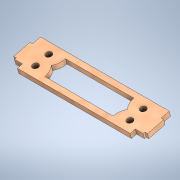
# Autodesk Inventor part: motor_holder
Saved by Autodesk Inventor 2022 (Build 260153070, 153G)
## iProperties
Created: 2021-05-28
Part Number: motor_holder
Material: Plywood, Sheathing, Glazed
Document SubType Name: Modeling
Designer: kardo
Density: 0.75 g/cm^3
Appearance: Plywood - New(2)
Author: kardo
Autodesk Inventor part; units mm, degrees
ref_plane "YZ Plane" through (0, 0, 0) normal (1, 0, 0) x (0, 1, 0)
ref_plane "XZ Plane" through (0, 0, 0) normal (0, 1, 0) x (-1, 0, 0)
ref_plane "XY Plane" through (0, 0, 0) normal (0, 0, 1) x (1, 0, 0)
derived "frame_outline.ipt"
sketch "motor_holder" plane through (6.24, -155.2, 37.8624) normal (0, 0.9709921, 0.2391117) x (-1, 0, 0)
  line L0 (-48.76, 5.318) -> (-48.76, -7.3978)
  line L1 (6.24, -320.5362) -> (6.24, 745.7309) construction
  line L2 (-48.76, 11.6759) -> (0.24, 11.6759)
  line L3 (-48.76, -13.7557) -> (0.24, -13.7557)
  line L4 (-48.76, 11.6759) -> (-48.76, 5.318)
  line L5 (-48.76, -7.3978) -> (-48.76, -13.7557)
  line L6 (0.24, 11.6759) -> (0.24, -13.7557)
  point P0 (6.24, -73.8742)
ref_plane "plane_shaft_perpendicular" through (6.24, -155.2, 37.8624) normal (0, 0.9709921, 0.2391117) x (-1, 0, 0)
sketch "Sketch7" plane through (6.24, -155.2, 37.8624) normal (0, 0.9709921, 0.2391117) x (-1, 0, 0)
  line L0 (-48.76, -7.3978) -> (-48.76, -13.7557) projected
  line L1 (-48.76, 5.318) -> (-48.76, -7.3978) projected
  line L2 (-48.76, 11.6759) -> (-48.76, 5.318) projected
  line L3 (0.24, 11.6759) -> (0.24, -13.7557) projected
  line L4 (-48.76, -13.7557) -> (0.24, -13.7557) projected
  line L5 (-48.76, 10.6759) -> (0.24, 10.6759)
  point P0 (6.24, -73.8742)
  dimension "d26" = 1
  constraints: 2 end point, 2 point on line, 1 parallel
  measures "d26" distance from line of L2.start L5
extrude "Extrusion5" add sketch "Sketch7" against normal blind 4
sketch "Sketch2" plane through (6, -151.9108, 24.5057) normal (0, 0.9709921, 0.2391117) x (1, 0, 0)
  line L0 (49, -19.0737) -> (51, -19.0737)
  line L1 (51, -19.0737) -> (51, -6.3579)
  line L2 (51, -6.3579) -> (49, -6.3579)
  line L3 (49, -19.0737) -> (49, -6.3579) projected
  point P0 (-6, 60.1185)
  dimension "d29" = 2
  constraints: 6 end point, 2 perpendicular, 1 parallel
  measures "d29" distance between parallel lines of L3 L1
extrude "Extrusion2" add sketch "Sketch2" against normal up to surface (4 mm away)
sketch "Sketch3" plane through (6, -151.9108, 24.5057) normal (0, 0.9709921, 0.2391117) x (1, 0, 0)
  line L0 (49, -20.4316) -> (43, -20.4316)
  line L1 (43, -20.4316) -> (43, -24.4316)
  line L2 (49, -24.4316) -> (49, -19.0737) projected
  line L3 (0, -24.4316) -> (49, -24.4316) projected
  point P0 (-6, 60.1185)
  dimension "d30" = 4
  dimension "d31" = 6
  constraints: 4 end point, 2 parallel, 2 point on line, 1 vertical
  measures "d30" distance of L0.end L1.end
  measures "d31" distance of L0.start L0.end
extrude "Extrusion3" cut sketch "Sketch3" against normal through all
sketch "Sketch5" plane through (6, -151.9108, 24.5057) normal (0, 0.9709921, 0.2391117) x (1, 0, 0)
  line L0 (0, -20.3597) -> (29, -20.3597)
  line L1 (29, -20.3597) -> (29, -4.0719) construction
  line L2 (29, -4.0719) -> (0, -4.0719)
  arc A0 (29, -12.2158) -> (25.946, -20.3597) centre (38.3315, -20.3597) ccw
  arc A1 (25.946, -4.0719) -> (29, -12.2158) centre (38.3315, -4.0719) ccw
  line L3 (25.946, -20.3597) -> (25.946, -4.0719) construction
  line L4 (0, -24.4316) -> (43, -24.4316) projected
  line L5 (43, -24.4316) -> (43, -20.4316) projected
  line L6 (0, 0) -> (0, -24.4316) projected
  line L7 (49, 0) -> (0, 0) projected
  point P0 (-6, 60.1185)
  dimension "d25" = 3.0539
  dimension "d32" = 24.4316
  dimension "d33" = 4.0719
  dimension "d34" = 4.0719
  dimension "d35" = 14
  constraints: 8 end point, 6 point on line, 4 parallel, 4 point on circle, 2 centre point, 1 midpoint
  measures "d25" distance between parallel lines of L1 L3
  measures "d32" distance of L6.start L4.start
  measures "d33" distance between parallel lines of L4 L0
  measures "d34" distance between parallel lines of L7 L2
  measures "d35" distance between parallel lines of L5 L1
extrude "Extrusion4" cut sketch "Sketch5" against normal through all
sketch "Sketch6" plane through (6, -151.9108, 24.5057) normal (0, 0.9709921, 0.2391117) x (1, 0, 0)
  line L0 (36, -17.4316) -> (36, -7) construction
  line L1 (43, -12.2158) -> (36, -12.2158) construction
  line L2 (36, -17.4316) -> (36, -24.4316) construction
  line L3 (36, -12.2158) -> (29, -12.2158) construction
  line L4 (36, -7) -> (36, 0) construction
  line L5 (0, -24.4316) -> (43, -24.4316) projected
  line L6 (49, 0) -> (0, 0) projected
  line L7 (43, -24.4316) -> (43, -20.4316) projected
  point P0 (-6, 60.1185)
  dimension "d36" = 7
  constraints: 10 end point, 4 collinear, 3 perpendicular, 3 point on line, 1 coincident, 1 midpoint
  measures "d36" distance from line of L5 L0.start
hole "Hole1" at (42, -156.079, 41.4317) at (42, -153.5846, 31.3026) direction (0, -0.9709921, -0.2391117) diameter 4.5 end through all
mirror "Mirror2" about plane through (6, -157.7527, 48.2286) normal (-1, 0, 0)
equation "\"d26\" = cowl_insulation_thickness - cowl_liner_thickness"
equation "\"d27\" = 2 * bulkhead_thickness"
equation "\"d29\" = bulkhead_thickness"
equation "\"d30\" = 2 * cowl_liner_thickness"
equation "\"d31\" = cowl_insulation_width"
equation "\"d25\" = 0.125 * d32"
equation "\"d33\" = 0.166667 * d32"
equation "\"d34\" = 0.166667 * d32"
equation "\"cowl_insulation_thickness\" = 3"
equation "\"cowl_liner_thickness\" = 2"
equation "\"bulkhead_thickness\" = 2"
equation "\"cowl_insulation_width\" = 6"
body "Solid1"
